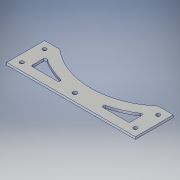
# Autodesk Inventor part: Upper Cross Bracket
Saved by Autodesk Inventor 2020.2 (Build 242310000, 310)
## iProperties
Created: 2019-03-23
Part Number: Upper Cross Bracket
Material: Aluminum 6061
Document SubType Name: Modeling
Designer: Richard Hall
Density: 2.7 g/cm^3
Appearance: Aluminum - Flat
Author: Richard Hall
Autodesk Inventor part; units mm, degrees
ref_plane "YZ Plane" through (0, 0, 0) normal (1, 0, 0) x (0, 1, 0)
ref_plane "XZ Plane" through (0, 0, 0) normal (0, 1, 0) x (-1, 0, 0)
ref_plane "XY Plane" through (0, 0, 0) normal (0, 0, 1) x (1, 0, 0)
sketch "Sketch1" plane through (0, 0, 0) normal (0, 1, 0) x (-1, 0, 0)
  line L0 (85, -50) -> (65, -50)
  line L1 (-85, -50) -> (-85, 0)
  line L2 (-85, 0) -> (85, 0)
  line L3 (85, 0) -> (85, -50)
  line L4 (85, -50) -> (-85, 0) construction
  line L5 (-85, -50) -> (85, 0) construction
  arc A0 (65, -50) -> (-65, -50) centre (0, -126.0208) ccw
  line L6 (65, -50) -> (-65, -50) construction
  line L7 (-65, -50) -> (-85, -50)
  line L8 (65, -28.5948) -> (65, -14)
  line L9 (63, -12) -> (30.2021, -12)
  arc A1 (61.914, -30.2742) -> (29.6815, -15.931) centre (0, -126.0208) ccw
  line L10 (0, 0) -> (0, -25)
  arc A2 (30.2021, -12) -> (29.6815, -15.931) centre (30.2021, -14) ccw
  arc A3 (65, -14) -> (63, -12) centre (63, -14) ccw
  arc A4 (61.914, -30.2742) -> (65, -28.5948) centre (63, -28.5948) ccw
  line L11 (-65, -28.5948) -> (-65, -14)
  line L12 (-63, -12) -> (-30.2021, -12)
  arc A5 (-29.6815, -15.931) -> (-61.914, -30.2742) centre (0, -126.0208) ccw
  arc A6 (-29.6815, -15.931) -> (-30.2021, -12) centre (-30.2021, -14) ccw
  arc A7 (-63, -12) -> (-65, -14) centre (-63, -14) ccw
  arc A8 (-65, -28.5948) -> (-61.914, -30.2742) centre (-63, -28.5948) ccw
  point P0 (0, -25)
  point P1 (0, -25)
  point P2 (65, -32.3419)
  point P3 (0, -12)
  dimension "d0" = 170
  dimension "d1" = 50
  dimension "d2" = 26
  dimension "d3" = 20
  dimension "d4" = 12
  dimension "d5" = 20
  dimension "d6" = 2
  constraints: 26 end point, 20 point on circle, 9 centre point, 9 symmetric about line, 7 tangent, 5 midpoint, 4 parallel, 4 perpendicular, 3 horizontal, 3 point on line, 2 equal radius, 2 vertical, 1 coincident, 1 concentric, 1 vertical alignment, 4 other
  measures "d0" distance of L1.end L2.end
  measures "d1" distance of L1.start L1.end
  measures "d2" distance edge to line of A0 L2
  measures "d3" distance from line of L3 L0.end
  measures "d4" distance between parallel lines of L2 L9
  measures "d5" distance between parallel lines of L3 L8
  measures "d6" radius of A2
extrude "Extrusion1" add sketch "Sketch1" along normal mid plane 3.175
sketch "Sketch2" plane through (0, 1.5875, 0) normal (0, 1, 0) x (1, 0, 0)
  line L0 (-85, 0) -> (85, 0) projected
  line L1 (-85, 50) -> (-85, 0) projected
  line L2 (-65, 50) -> (-85, 50) projected
  line L3 (0, 0) -> (0, 15.0505)
  point P0 (-75, 10)
  point P1 (-75, 40)
  point P2 (75, 10)
  point P3 (75, 40)
  dimension "d9" = 10
  dimension "d10" = 10
  dimension "d11" = 10
  constraints: 2 end point, 2 symmetric about line, 1 vertical, 1 vertical alignment
  measures "d9" distance from line of L0 point (-75, 10)
  measures "d10" distance from line of L1 point (-75, 10)
  measures "d11" distance from line of L2 point (-75, 40)
hole "Hole1" at (-75, 1.5875, -10) at (-75, 1.5875, -40) at (75, 1.5875, -40) at (75, 1.5875, -10) direction (0, -1, 0) diameter 5 end through all clearance for "Flat Head Machine Screw" size "M5" standard "Ansi Metric M Profile"
sketch "Sketch4" plane through (0, 1.5875, 0) normal (0, 1, 0) x (1, 0, 0)
  line L0 (-85, 50) -> (-85, 0) projected
  arc A0 (-30.2021, 12) -> (-29.6815, 15.931) centre (-30.2021, 14) ccw projected
  line L1 (-85, 0) -> (85, 0) projected
  point P0 (0, 0)
  point P1 (-5, 10)
  dimension "d29" = 80
  dimension "d37" = 10
  measures "d29" distance from line of point (-5, 10) L0
  measures "d37" distance from line of L1 point (-5, 10)
hole "Hole3" at (-5, 1.5875, -10) direction (0, -1, 0) diameter 5.5118 depth 14.2 tip angle 118 clearance for "Socket Head Cap Screw" size "M5" standard "Ansi Metric M Profile"
body "Solid1"
